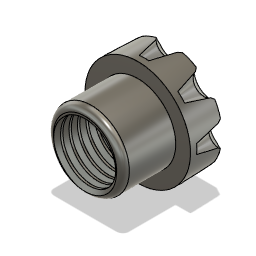
InnerFeeder_Cap_T1 (Autodesk Fusion 360 design; units mm, degrees)
Autodesk Fusion 360 part; units mm, degrees
sketch "Skizze1" plane through (0, 0, 0) normal (0, 1, 0) x (1, 0, 0)
  circle A0 centre (0, 0) radius 9
  dimension "d1" = 18
  constraint coincident A0.centre origin
  measures "d1" diameter of A0
extrude "Extrusion1" add sketch "Skizze1" along normal blind 12.5 makes body 1
sketch "Skizze2" plane through (0, 0, 0) normal (0, 1, 0) x (1, 0, 0)
  circle A0 centre (0, 0) radius 12.5
  dimension "d4" = 25
  constraint coincident A0.centre origin
  measures "d4" diameter of A0
extrude "Extrusion2" add sketch "Skizze2" along normal blind 8.5 separate body makes body 2
move_body "Verschieben1" bodies 1 to x (1, 0, 0) y (0, 1, 0) z (0, 0, 1) at (0, 8.5, 0)
sketch "Skizze4" plane through (0, 0, 0) normal (0, 1, 0) x (1, 0, 0)
  circle A0 centre (8.8385, -8.8385) radius 3
  circle A1 centre (12.5, 0) radius 3
  circle A2 centre (8.8439, 8.8439) radius 3
  circle A3 centre (0, 12.5) radius 3
  circle A4 centre (-12.5, 0) radius 3
  circle A5 centre (-8.8332, 8.8332) radius 3
  circle A6 centre (0, -12.5) radius 3
  circle A7 centre (-8.8378, -8.8378) radius 3
  dimension "d7" = 6
  dimension "d8" = 6
  dimension "d9" = 6
  dimension "d10" = 6
  dimension "d11" = 6
  dimension "d12" = 6
  dimension "d13" = 6
  dimension "d14" = 6
  measures "d7" diameter of A0
  measures "d8" diameter of A1
  measures "d9" diameter of A2
  measures "d10" diameter of A3
  measures "d11" diameter of A4
  measures "d12" diameter of A5
  measures "d13" diameter of A6
  measures "d14" diameter of A7
extrude "Extrusion3" cut sketch "Skizze4" along normal blind 7 draft -15 bodies 2
chamfer "Fase1" distance 1 angle 60 16 edges at (-4.7831, 0, -11.5487) (0, 0, -9.5) (4.7839, 0, -11.5483) (6.7226, 0, -6.7226) (9.5, 0, 0) (11.5483, 0, -4.7839) (11.5485, 0, 4.7835) (6.7172, 0, 6.7172) (4.7835, 0, 11.5485) (0, 0, 9.5) (-4.7835, 0, 11.5485) (-6.7165, 0, 6.7165) (-11.5485, 0, 4.7835) (-9.5, 0, 0) (-11.5487, 0, -4.7831) (-6.7119, 0, -6.7119) measured on face at (6.9335, 5.1667, -10.4008) measured on face at (0.0018, 0, 3.1684) measured on face at (6.9335, 5.1667, -10.4008) measured on face at (0.0018, 0, 3.1684) measured on face at (0.0018, 0, 3.1684) measured on face at (6.9335, 5.1667, -10.4008) measured on face at (6.9335, 5.1667, -10.4008) measured on face at (0.0018, 0, 3.1684) measured on face at (6.9335, 5.1667, -10.4008) measured on face at (0.0018, 0, 3.1684) measured on face at (6.9335, 5.1667, -10.4008) measured on face at (0.0018, 0, 3.1684) measured on face at (6.9335, 5.1667, -10.4008) measured on face at (0.0018, 0, 3.1684) measured on face at (6.9335, 5.1667, -10.4008) measured on face at (0.0018, 0, 3.1684) on bodies 2
sketch "Skizze7" plane through (0, 0, 0) normal (0, 1, 0) x (1, 0, 0)
  circle A0 centre (0, 0) radius 7.5
  constraint coincident A0.centre origin
move_body "Verschieben2" bodies 1 2 to x (1, 0, 0) y (0, 1, 0) z (0, 0, 1) at (0, -21, 0)
extrude "Extrusion4" cut sketch "Skizze7" against normal blind 19 bodies 1
sketch "Skizze8" plane through (0, 0, 0) normal (0, 1, 0) x (1, 0, 0)
  circle A0 centre (0, 0) radius 1.25
  dimension "d22" = 2.5
  constraint coincident A0.centre origin
  measures "d22" diameter of A0
extrude "Extrusion5" cut sketch "Skizze8" against normal blind 32 bodies 2
thread "Gewinde1" "ISO Metric profile 16.0 M16x2 6H" major diameter 16.2505 minor diameter 14.0225 pitch 2 angle 60 modelled right hand crest width 0.5471 on face at (7.4627, -4.1667, 0.7468) from (0, 0, 0) to (0, -12.5, 0) crest through (7.0113, -0.5, 0) on bodies 1
fillet "Abrundung1" radius 1.5 1 edges at (-8.3909, 0, 3.2545) on bodies 1
move_body "Verschieben3" bodies 1 2 to x (1, 0, 0) y (0, 0, 1) z (0, -1, 0) at (0, -22.1432, 4.1432)
